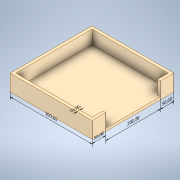
# Autodesk Inventor part: 放书的
Saved by Autodesk Inventor 2020 (Build 240168000, 168)
## iProperties
Created: 2021-04-04
Part Number: 放书的
Material: 聚乙烯，低密度
Document SubType Name: Modeling
Designer: 70929
Density: 0.894 g/cm^3
Appearance: 平滑 - 灰白色
Author: 70929
Autodesk Inventor part; units mm, degrees
ref_plane "YZ Plane" through (0, 0, 0) normal (1, 0, 0) x (0, 1, 0)
ref_plane "XZ Plane" through (0, 0, 0) normal (0, 1, 0) x (-1, 0, 0)
ref_plane "XY Plane" through (0, 0, 0) normal (0, 0, 1) x (1, 0, 0)
sketch "草图1" plane through (0, 0, 0) normal (0, 1, 0) x (-1, 0, 0)
  line L0 (150, 150) -> (-150, 150)
  line L1 (-150, 150) -> (-150, -150)
  line L2 (-150, -150) -> (150, -150)
  line L3 (150, -150) -> (150, 150)
  line L4 (150, 150) -> (-150, -150) construction
  line L5 (-150, 150) -> (150, -150) construction
  point P0 (0, 0)
  dimension "d0" = 300
  dimension "d1" = 300
  constraints: 12 end point, 2 midpoint, 2 parallel, 1 horizontal, 1 perpendicular
  measures "d0" distance of L2.end L1.end
  measures "d1" distance of L0.end L1.end
extrude "拉伸1" add sketch "草图1" along normal blind 10
sketch "草图3" plane through (0, 10, 0) normal (0, 1, 0) x (1, 0, 0)
  line L0 (-150, -150) -> (-150, 150) projected
  line L1 (-150, 150) -> (150, 150) projected
  line L2 (150, 150) -> (150, -150) projected
  line L3 (150, -150) -> (-150, -150) projected
  line L4 (-140, -140) -> (-140, 140)
  line L5 (-140, 140) -> (140, 140)
  line L6 (140, 140) -> (140, -140)
  line L7 (140, -140) -> (-140, -140)
  point P0 (0, 0)
  dimension "d5" = 10
  constraints: 8 end point, 3 other
  measures "d5" distance between parallel lines of L3 L7
extrude "拉伸2" add sketch "草图3" along normal blind 50
sketch "草图4" plane through (150, 0, 150) normal (1, 0, 0) x (0, 0, -1)
  line L0 (0, 60) -> (300, 60) projected
  line L1 (300, 60) -> (300, 0) projected
  line L2 (300, 0) -> (0, 0) projected
  line L3 (0, 0) -> (0, 60) projected
  line L4 (0, 0) -> (0, 60) projected
  line L5 (0, 60) -> (50, 60)
  line L6 (300, 60) -> (0, 60) projected
  line L7 (300, 60) -> (250, 60)
  line L8 (50, 60) -> (50, 10)
  line L9 (300, 0) -> (0, 0) projected
  line L10 (250, 60) -> (250, 10)
  line L11 (290, 10) -> (10, 10) projected
  line L12 (50, 10) -> (250, 10)
  point P0 (150, 0)
  point P1 (250, 0)
  point P2 (250, 60)
  point P3 (53, 0)
  dimension "d8" = 300
  dimension "d9" = 50
  dimension "d18" = 50
  constraints: 10 end point, 5 point on line, 2 perpendicular
  measures "d8" distance of L0.start L0.end
  measures "d9" distance of L0.end L7.end
  measures "d18" distance between parallel lines of L3 L8
extrude "拉伸3" cut sketch "草图4" against normal blind 10 contours L0 L10 L11 L8
